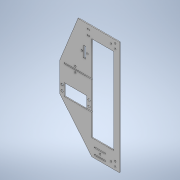
# Autodesk Inventor part: SIdeFinal
Saved by Autodesk Inventor 2020 (Build 240168000, 168)
## iProperties
Created: 2019-06-17
Part Number: SIdeFinal
Material: Generic
Document SubType Name: Modeling
Designer: Vivek Muskan
Density: 1 g/cm^3
Appearance: Default
Author: Vivek Muskan
Autodesk Inventor part; units mm, degrees
ref_plane "YZ Plane" through (0, 0, 0) normal (1, 0, 0) x (0, 1, 0)
ref_plane "XZ Plane" through (0, 0, 0) normal (0, 1, 0) x (-1, 0, 0)
ref_plane "XY Plane" through (0, 0, 0) normal (0, 0, 1) x (1, 0, 0)
sketch "Sketch1" plane through (0, 0, 0) normal (0, 0, 1) x (1, 0, 0)
  line L0 (95, 60) -> (105, 60)
  line L1 (105, 60) -> (105, 10)
  line L2 (105, 10) -> (100, 10)
  line L3 (100, 10) -> (100, 20)
  line L4 (100, 20) -> (95, 20)
  line L5 (95, 20) -> (95, 60)
  line L6 (105, -60) -> (95, -60)
  line L7 (95, -60) -> (95, -20)
  line L8 (95, -20) -> (100, -20)
  line L9 (100, -20) -> (100, -10)
  line L10 (100, -10) -> (105, -10)
  line L11 (105, -10) -> (105, -60)
  line L12 (120.5, 3.5) -> (123.5, 3.5)
  line L13 (123.5, 3.5) -> (123.5, 5)
  line L14 (123.5, 5) -> (127, 5)
  line L15 (127, 5) -> (127, -5)
  line L16 (127, -5) -> (123.5, -5)
  line L17 (123.5, -5) -> (123.5, -3.5)
  line L18 (123.5, -3.5) -> (120.5, -3.5)
  line L19 (120.5, -3.5) -> (120.5, -5)
  line L20 (120.5, -5) -> (117, -5)
  line L21 (117, -5) -> (117, -49)
  line L22 (117, -49) -> (107, -51)
  line L23 (107, -51) -> (107, -10)
  line L24 (107, -10) -> (112, -10)
  line L25 (112, -10) -> (112, -3.5)
  line L26 (112, -3.5) -> (100, -3.5)
  line L27 (100, -3.5) -> (100, -4)
  line L28 (100, -4) -> (45, -4)
  arc A0 (43, -6) -> (45, -4) centre (43, -4) ccw
  line L29 (43, -6) -> (42, -6)
  arc A1 (40, -4) -> (42, -6) centre (42, -4) ccw
  line L30 (40, -4) -> (5, -4)
  arc A2 (3, -6) -> (5, -4) centre (3, -4) ccw
  line L31 (3, -6) -> (2, -6)
  arc A3 (0, -4) -> (2, -6) centre (2, -4) ccw
  line L32 (0, -4) -> (0, 4)
  arc A4 (2, 6) -> (0, 4) centre (2, 4) ccw
  line L33 (2, 6) -> (3, 6)
  arc A5 (5, 4) -> (3, 6) centre (3, 4) ccw
  line L34 (5, 4) -> (40, 4)
  arc A6 (42, 6) -> (40, 4) centre (42, 4) ccw
  line L35 (42, 6) -> (43, 6)
  arc A7 (45, 4) -> (43, 6) centre (43, 4) ccw
  line L36 (45, 4) -> (100, 4)
  line L37 (100, 4) -> (100, 3.5)
  line L38 (100, 3.5) -> (112, 3.5)
  line L39 (112, 3.5) -> (112, 10)
  line L40 (112, 10) -> (107, 10)
  line L41 (107, 10) -> (107, 51)
  line L42 (107, 51) -> (117, 49)
  line L43 (117, 49) -> (117, 5)
  line L44 (117, 5) -> (120.5, 5)
  line L45 (120.5, 5) -> (120.5, 3.5)
  line L46 (92, 27.5) -> (92, 26)
  line L47 (92, 26) -> (42, 26)
  line L48 (42, 26) -> (42, 27.5)
  line L49 (42, 27.5) -> (92, 27.5)
  line L50 (92, -24) -> (92, -25.5)
  line L51 (92, -25.5) -> (42, -25.5)
  line L52 (42, -25.5) -> (42, -24)
  line L53 (42, -24) -> (92, -24)
  line L54 (92, -25.5) -> (82, -25.5)
  line L55 (82, -25.5) -> (82, -24)
  line L56 (82, -24) -> (77, -24)
  line L57 (77, -24) -> (77, -25.5)
  line L58 (77, -25.5) -> (57, -25.5)
  line L59 (57, -25.5) -> (57, -24)
  line L60 (57, -24) -> (52, -24)
  line L61 (52, -24) -> (52, -25.5)
  line L62 (52, -25.5) -> (42, -25.5)
  line L63 (42, -25.5) -> (42, 27.5)
  line L64 (92, 27.5) -> (92, 97.5)
  line L65 (92, -25.5) -> (92, -65.5)
  line L66 (92, -65.5) -> (132, -65.5)
  line L67 (132, -65.5) -> (142, -65.5)
  line L68 (132, -65.5) -> (132, 97.5)
  line L69 (142, -65.5) -> (142, 109.5)
  line L70 (42, 27.5) -> (34, 27.5)
  line L71 (95, 60) -> (105, 60)
  line L72 (105, 60) -> (105, 84)
  line L73 (105, 84) -> (95, 84)
  line L74 (95, 84) -> (95, 60)
  line L75 (95, 60) -> (95, 90)
  line L76 (95, 90) -> (132, 90)
  line L77 (95, 90) -> (92, 90)
  line L78 (142, -65.5) -> (142, -95.5)
  line L79 (142, -95.5) -> (92, -95.5)
  line L80 (92, -95.5) -> (34, -25.5)
  line L81 (34, -25.5) -> (34, 27.5)
  line L82 (0, 0) -> (71, 0)
  line L83 (23.8389, -219.7015) -> (66.8389, -219.7015)
  line L84 (66.8389, -219.7015) -> (66.8389, -198.7015)
  line L85 (66.8389, -198.7015) -> (23.8389, -198.7015)
  line L86 (23.8389, -198.7015) -> (23.8389, -219.7015)
  line L87 (45.3389, -198.7015) -> (45.3389, -219.7015)
  line L88 (66.8389, -198.7015) -> (66.8389, -203.7015)
  line L89 (66.8389, -203.7015) -> (70.8389, -203.7015)
  line L90 (70.8389, -203.7015) -> (70.8389, -213.7015)
  circle A8 centre (70.8389, -213.7015) radius 2
  circle A9 centre (70.8389, -203.7015) radius 2
  line L91 (66.8389, -209.2015) -> (56.8389, -209.2015)
  line L92 (56.8389, -209.2015) -> (56.8389, -189.2015)
  line L93 (56.8389, -189.2015) -> (56.8389, -229.2015)
  circle A10 centre (19.8389, -213.7015) radius 2
  circle A11 centre (19.8389, -203.7015) radius 2
  line L94 (33.8389, -189.2015) -> (33.8389, -229.2015)
  line L95 (42, -24) -> (83, -24)
  line L96 (83, -24) -> (83, -4)
  line L97 (83, -4) -> (42, -4)
  line L98 (42, -4) -> (42, -24)
  line L99 (62.5, -4) -> (62.5, -24)
  line L100 (83, -4) -> (83, -9)
  line L101 (83, -9) -> (87, -9)
  line L102 (87, -9) -> (87, -19)
  circle A12 centre (87, -9) radius 2
  circle A13 centre (87, -19) radius 2
  circle A14 centre (38, -9) radius 2
  circle A15 centre (38, -19) radius 2
  line L103 (92, -24) -> (92, 26)
  line L104 (109.5, -120.7576) -> (69.5, -120.7576)
  line L105 (69.5, -120.7576) -> (69.5, 125.4146)
  line L106 (142, 109.5) -> (67, 109.5)
  line L107 (67, 109.5) -> (67, 109.5)
  line L108 (67, 109.5) -> (34, 27.5)
  line L109 (34, 27.5) -> (69.5, 27.5)
  line L110 (69.5, 27.5) -> (69.5, 52.5)
  line L111 (92, 27.5) -> (69.5, 27.5)
  line L112 (92, 27.5) -> (77, 27.5)
  line L113 (77, 27.5) -> (77, 52.5)
  line L114 (77, 52.5) -> (78.5, 52.5)
  line L115 (78.5, 72.5) -> (77, 72.5)
  line L116 (77, 72.5) -> (77, 52.5)
  line L117 (78.5, 52.5) -> (81, 52.5)
  line L118 (81, 52.5) -> (81, 72.5)
  line L119 (81, 72.5) -> (78.5, 72.5)
  line L120 (81, 62.5) -> (79, 62.5)
  line L121 (79, 62.5) -> (74, 62.5)
  line L122 (74, 62.5) -> (84, 62.5)
  circle A16 centre (74, 62.5) radius 1.5
  circle A17 centre (84, 62.5) radius 1.5
  line L123 (92, -95.5) -> (92, -90.5)
  line L124 (92, -90.5) -> (97, -90.5)
  line L125 (97, -90.5) -> (117, -90.5)
  line L126 (117, -90.5) -> (117, -89)
  line L127 (117, -89) -> (97, -89)
  line L128 (97, -89) -> (97, -90.5)
  line L129 (97, -89) -> (97, -79)
  line L130 (97, -79) -> (117, -79)
  line L131 (117, -79) -> (117, -77.5)
  line L132 (117, -77.5) -> (97, -77.5)
  line L133 (97, -77.5) -> (97, -79)
  line L134 (107, -90.5) -> (107, -84)
  circle A18 centre (107, -84) radius 1.5
  point P0 (59.5188, -93.2152)
  point P1 (83, -4)
  point P2 (83, -24)
  dimension "d0" = 10
  dimension "d1" = 1.5
  dimension "d2" = 5
  dimension "d3" = 1.5
  dimension "d4" = 20
  dimension "d5" = 1.5
  dimension "d6" = 5
  dimension "d7" = 1.5
  dimension "d8" = 70
  dimension "d9" = 40
  dimension "d10" = 40
  dimension "d11" = 40
  dimension "d12" = 10
  dimension "d13" = 175
  dimension "d14" = 8
  dimension "d15" = 10
  dimension "d16" = 24
  dimension "d17" = 30
  dimension "d19" = 30
  dimension "d20" = 50
  dimension "d21" = 71
  dimension "d22" = 43
  dimension "d23" = 21
  dimension "d24" = 5
  dimension "d25" = 4
  dimension "d26" = 10
  dimension "d27" = 4
  dimension "d28" = 4
  dimension "d29" = 10
  dimension "d30" = 20
  dimension "d31" = 40
  dimension "d32" = 41
  dimension "d33" = 20
  dimension "d34" = 5
  dimension "d35" = 4
  dimension "d36" = 10
  dimension "d37" = 4
  dimension "d38" = 4
  dimension "d48" = 40
  dimension "d49" = 3
  dimension "d50" = 75
  dimension "d51" = 0
  dimension "d62" = 15
  dimension "d63" = 25
  dimension "d64" = 1.5
  dimension "d65" = 20
  dimension "d73" = 2.5
  dimension "d74" = 2
  dimension "d75" = 5
  dimension "d76" = 10
  dimension "d77" = 3
  dimension "d78" = 3
  dimension "d81" = 5
  dimension "d82" = 5
  dimension "d83" = 20
  dimension "d84" = 1.5
  dimension "d85" = 10
  dimension "d86" = 20
  dimension "d87" = 1.5
  dimension "d88" = 3
  constraints: 270 end point, 22 point on line, 20 perpendicular, 19 centre point, 16 parallel, 16 point on circle, 12 horizontal, 7 coincident, 7 midpoint, 6 symmetric about line, 6 vertical, 2 collinear, 4 other
  measures "d0" distance of L50.end L54.end
  measures "d1" distance of L54.end L55.end
  measures "d2" distance of L55.end L56.end
  measures "d3" distance of L56.end L57.end
  measures "d4" distance of L57.end L58.end
  measures "d5" distance of L58.end L59.end
  measures "d6" distance of L59.end L60.end
  measures "d7" distance of L60.end L61.end
  measures "d8" distance of L46.start L64.end
  measures "d9" distance of L64.end L68.end
  measures "d10" distance of L50.end L65.end
  measures "d11" distance of L65.end L66.end
  measures "d12" distance of L66.end L67.end
  measures "d13" distance of L67.end L69.end
  measures "d14" distance of L48.end L70.end
  measures "d15" distance of L73.end L72.end
  measures "d16" distance of L72.end L71.end
  measures "d17" distance of L0.start L75.end
  measures "d19" distance of L67.end L78.end
  measures "d20" distance of L78.end L79.end
  measures "d21" distance of L82.start L82.end
  measures "d22" distance of L85.end L84.end
  measures "d23" distance of L84.end L83.end
  measures "d24" distance of L84.end L88.end
  measures "d25" distance of L88.end L89.end
  measures "d26" distance of L89.end L90.end
  measures "d27" diameter of A8
  measures "d28" diameter of A9
  measures "d29" distance of L91.start L91.end
  measures "d30" distance of L91.end L92.end
  measures "d31" distance of L92.end L93.end
  measures "d32" distance of L97.end L96.end
  measures "d33" distance of L96.end L95.end
  measures "d34" distance of L96.end L100.end
  measures "d35" distance of L100.end L101.end
  measures "d36" distance of L101.end L102.end
  measures "d37" diameter of A12
  measures "d38" diameter of A13
  measures "d48" distance of L104.start L104.end
  measures "d49" distance of L75.end L77.end
  measures "d50" distance of L69.end L106.end
  measures "d51" distance of L106.end L107.end
  measures "d62" distance of L46.start L112.end
  measures "d63" distance of L112.end L113.end
  measures "d64" distance of L115.end L115.start
  measures "d65" distance of L115.start L114.end
  measures "d73" distance of L119.end L118.end
  measures "d74" distance of L120.start L120.end
  measures "d75" distance of L120.end L121.end
  measures "d76" distance of L121.end L122.end
  measures "d77" diameter of A16
  measures "d78" diameter of A17
  measures "d81" distance of L79.end L123.end
  measures "d82" distance of L123.end L124.end
  measures "d83" distance of L127.end L126.end
  measures "d84" distance of L126.end L125.end
  measures "d85" distance of L127.end L129.end
  measures "d86" distance of L132.end L131.end
  measures "d87" distance of L131.end L130.end
  measures "d88" diameter of A18
extrude "Extrusion1" add sketch "Sketch1" along normal blind 1.5 contours A16 | A17 | L116 L121 L120 L118 L117 L114 | L77 L64 L49 L105 L106 L69 L67 L68 L76 | L133 L132 L131 L130 | A18 | L128 L127 L134 L125 | L67 L78 L79 L80 L105 L51 L65 L66 | L103 L36 L105 L47 | L105 L36 A7 L35 L63 L47 | L103 L28 L105 L36 | L49 L70 L108 L106 L105 | L53 L96 L28 L103 | L63 A6 L34 L81 L70 L48 | L105 L82 L63 L35 A7 L36 | L116 L115 L119 L118 L120 L121 | L80 L81 L30 A1 L63 L52 L51 L105 | L63 L82 L81 L34 A6 | L105 L28 L97 L63 L82 | L63 A1 L30 L81 L82 | L134 L127 L126 L125
sketch "Sketch2" plane through (0, 0, 1.5) normal (0, 0, 1) x (1, 0, 0)
  line L0 (42, 26) -> (42, 27.5) projected
  line L1 (42, 26.75) -> (62, 26.75)
  line L2 (62, 26.75) -> (62, 31.75)
  line L3 (62, 31.75) -> (62, 21.75)
  circle A0 centre (62, 31.75) radius 1.5
  circle A1 centre (62, 21.75) radius 1.5
  point P0 (0, 0)
  dimension "d41" = 20
  dimension "d42" = 5
  dimension "d43" = 10
  dimension "d44" = 3
  dimension "d45" = 3
  constraints: 6 end point, 2 centre point, 2 coincident, 1 horizontal, 1 midpoint, 1 perpendicular, 1 point on line
  measures "d41" distance of L1.start L1.end
  measures "d42" distance of L1.end L2.end
  measures "d43" distance of L2.end L3.end
  measures "d44" diameter of A0
  measures "d45" diameter of A1
extrude "Extrusion2" cut sketch "Sketch2" against normal blind 1.5
extrude "Extrusion5" cut sketch "Sketch1" along normal blind 1.5 contours A16 | A17 | L116 L121 L120 L118 L117 L114 | L116 L115 L119 L118 L120 L121
extrude "Extrusion6" cut sketch "Sketch1" along normal blind 1.5 contours L133 L132 L131 L130 | A18 | L128 L127 L134 L125 | L134 L127 L126 L125
sketch "Sketch3" plane through (0, 0, 1.5) normal (0, 0, 1) x (1, 0, 0)
  line L0 (81, 72.5) -> (81, 52.5) projected
  line L1 (81, 72.5) -> (81, 102.5)
  line L2 (42, 27.5) -> (92, 27.5) projected
  line L3 (81, 102.5) -> (81, 92.5)
  line L4 (81, 102.5) -> (83.5, 102.5)
  line L5 (83.5, 102.5) -> (83.5, 92.5)
  line L6 (83.5, 102.5) -> (88.5, 102.5)
  line L7 (88.5, 102.5) -> (88.5, 101)
  line L8 (88.5, 101) -> (83.5, 101)
  line L9 (83.5, 101) -> (83.5, 102.5)
  line L10 (83.5, 92.5) -> (88.5, 92.5)
  line L11 (88.5, 92.5) -> (88.5, 91)
  line L12 (88.5, 91) -> (83.5, 91)
  line L13 (83.5, 91) -> (83.5, 92.5)
  point P0 (0, 0)
  dimension "d93" = 30
  dimension "d94" = 10
  dimension "d95" = 2.5
  dimension "d96" = 5
  dimension "d97" = 1.5
  dimension "d98" = 5
  dimension "d99" = 1.5
  constraints: 24 end point, 4 parallel, 3 horizontal, 3 perpendicular, 1 point on line, 1 vertical
  measures "d93" distance of L0.start L1.end
  measures "d94" distance of L1.end L3.end
  measures "d95" distance of L1.end L4.end
  measures "d96" distance of L7.end L8.end
  measures "d97" distance of L6.end L7.end
  measures "d98" distance of L11.end L12.end
  measures "d99" distance of L10.end L11.end
extrude "Extrusion7" cut sketch "Sketch3" against normal blind 1.5
sketch "Sketch4" plane through (0, 0, 1.5) normal (0, 0, 1) x (1, 0, 0)
  line L0 (142, -95.5) -> (142, 109.5) projected
  line L1 (142, 109.5) -> (142, 99.5)
  line L2 (142, 99.5) -> (132, 99.5)
  line L3 (132, 99.5) -> (127, 99.5)
  circle A0 centre (127, 99.5) radius 1.5
  circle A1 centre (134.5, 95.1699) radius 1.5
  circle A2 centre (134.5, 103.8301) radius 1.5
  line L4 (142, -95.5) -> (142, -85.5)
  line L5 (142, -85.5) -> (132, -85.5)
  line L6 (132, -85.5) -> (127, -85.5)
  circle A3 centre (127, -85.5) radius 1.5
  circle A4 centre (134.5, -89.8301) radius 1.5
  circle A5 centre (134.5, -81.1699) radius 1.5
  point P0 (0, 0)
  dimension "d102" = 10
  dimension "d103" = 10
  dimension "d104" = 5
  dimension "d105" = 3
  dimension "d108" = 360
  dimension "d110" = 10
  dimension "d111" = 10
  dimension "d112" = 5
  dimension "d113" = 3
  dimension "d116" = 360
  constraints: 12 end point, 6 centre point, 4 point on line, 2 coincident, 2 perpendicular, 14 other
  measures "d102" distance of L0.end L1.end
  measures "d103" distance of L1.end L2.end
  measures "d104" distance of L2.end L3.end
  measures "d105" diameter of A0
  measures "d110" distance of L0.start L4.end
  measures "d111" distance of L4.end L5.end
  measures "d112" distance of L5.end L6.end
  measures "d113" diameter of A3
extrude "Extrusion8" cut sketch "Sketch4" against normal blind 1.5
body "Solid1"
